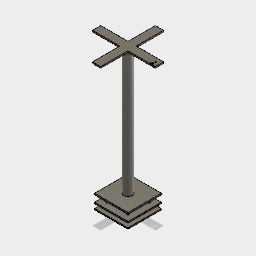
_FYP_Project.30689574-17b8-4f28-82bc-4a6d63cc6bb8 (Autodesk Fusion 360 design; units mm, degrees)
Autodesk Fusion 360 part; units mm, degrees
note: some values were not read from the file. Chosen so that the rebuilt part matches the saved one: which face or edge a step refers to. Set by a fixed rule: which sketch regions a step uses.
sketch "Sketch1" plane through (0, 0, 0) normal (1, 0, 0) x (0, 0, -1)
  circle A0 centre (0, 0) radius 40
  line L0 (-2.9, 1.75) -> (2.9, 1.75)
  line L1 (2.9, 1.75) -> (2.9, -1.75)
  line L2 (2.9, -1.75) -> (-2.9, -1.75)
  line L3 (-2.9, -1.75) -> (-2.9, 1.75)
  line L4 (-2.9, 1.75) -> (2.9, -1.75) construction
  line L5 (2.9, 1.75) -> (-2.9, -1.75) construction
  dimension "d1" = 80
  dimension "d2" = 5.8
  dimension "d3" = 3.5
  measures "d1" diameter of A0
  measures "d2" distance of L1.end L2.end
  measures "d3" distance of L0.end L1.end
sketch "Sketch2" plane through (0, 0, 0) normal (0, 1, 0) x (1, 0, 0)
  line L0 (16.6, 6) -> (-16.6, 6)
  line L1 (-16.6, 6) -> (-16.6, -6)
  line L2 (-16.6, -6) -> (16.6, -6)
  line L3 (16.6, -6) -> (16.6, 6)
  line L4 (16.6, 6) -> (-16.6, -6) construction
  line L5 (-16.6, 6) -> (16.6, -6) construction
  dimension "d6" = 33.2
  dimension "d7" = 12
  measures "d6" distance of L1.end L2.end
  measures "d7" distance of L0.end L1.end
extrude "Extrude2" add sketch "Sketch2" along normal blind 10 makes body 1
sketch "Sketch3" plane through (16.6, 0, 0) normal (1, 0, 0) x (0, 0, -1)
  line L0 (-6, 0) -> (6, 0)
  line L1 (6, 0) -> (6, 10)
  line L2 (6, 10) -> (-6, 10)
  line L3 (-6, 10) -> (-6, 0)
  circle A0 centre (-0.0016, 5.0186) radius 1.5
  line L4 (-1.2598, 5.8353) -> (1.2566, 5.8353)
  dimension "d10" = 3
  measures "d10" diameter of A0
extrude "Extrude3" add sketch "Sketch3" along normal blind 15 contours A0 L4 picked at (0.569, 4.736) bodies 1
sketch "Sketch4" plane through (0, 0, 0) normal (1, 0, 0) x (0, 0, -1)
  circle A0 centre (0, 0) radius 30
  dimension "d13" = 60
  measures "d13" diameter of A0
extrude "Extrude4" add sketch "Sketch4" along normal blind 8 separate body makes body 2
sketch "Sketch5" plane through (0, 0, 0) normal (-1, 0, 0) x (0, 0, 1)
  circle A0 centre (0, 0) radius 30
  circle A1 centre (0, 0) radius 1.5
  line L0 (-1.26, 0.8139) -> (1.26, 0.8139)
  dimension "d20" = 3
  dimension "d21" = 2.52
  measures "d20" diameter of A1
  measures "d21" distance of L0.start L0.end
extrude "Extrude5" cut sketch "Sketch5" against normal blind 14 contours A1 L0 picked at (-0.4465, 0.3176) bodies 2
copy_body "Body->Comp1" bodies 2 removing the originals makes body 3 in component "Component"
sketch "Sketch6" plane through (0, 0, 0) normal (0, 1, 0) x (1, 0, 0)
  line L0 (75, 100) -> (-75, 100)
  line L1 (-75, 100) -> (-75, -100)
  line L2 (-75, -100) -> (75, -100)
  line L3 (75, -100) -> (75, 100)
  line L4 (75, 100) -> (-75, -100) construction
  line L5 (-75, 100) -> (75, -100) construction
  dimension "d24" = 200
  dimension "d25" = 150
  measures "d24" distance of L0.end L1.end
  measures "d25" distance of L1.end L2.end
extrude "Extrude6" add sketch "Sketch6" along normal blind 6 separate body makes body 4
sketch "Sketch7" plane through (0, 6, 0) normal (0, 1, 0) x (-1, 0, 0)
  line L0 (-75, 100) -> (-75, -100)
  line L1 (-75, -100) -> (75, -100)
  line L2 (75, -100) -> (75, 100)
  line L3 (75, 100) -> (-75, 100)
  line L4 (-75, 38) -> (-41.8, 38)
  line L5 (-41.8, 38) -> (-41.8, 50)
  line L6 (-41.8, 50) -> (-75, 50)
  line L7 (-75, 50) -> (-75, 38)
  line L8 (-50.1369, 50) -> (-50.1369, 100)
  line L9 (75, 50) -> (41.8, 50)
  line L10 (41.8, 50) -> (41.8, 38)
  line L11 (41.8, 38) -> (75, 38)
  line L12 (75, 38) -> (75, 50)
  line L13 (63.0151, 50) -> (63.0151, 100)
  dimension "d28" = 33.2
  dimension "d29" = 12
  dimension "d30" = 50
  dimension "d31" = 33.2
  dimension "d32" = 12
  dimension "d33" = 50
  measures "d28" distance of L4.start L4.end
  measures "d29" distance of L4.start L6.end
  measures "d30" distance of L8.start L8.end
  measures "d31" distance of L9.start L9.end
  measures "d32" distance of L9.start L11.end
  measures "d33" distance of L13.start L13.end
extrude "Extrude7" add sketch "Sketch7" along normal blind 10 contours L0 L4 L5 L6 L7 | L2 L9 L10 L11 L12 bodies 4
sketch "Sketch8" plane through (75, 0, 0) normal (1, 0, 0) x (0, 0, -1)
  line L0 (-100, 0) -> (100, 0)
  line L1 (100, 0) -> (100, 6)
  line L2 (100, 6) -> (-38, 6)
  line L3 (-38, 6) -> (-38, 16)
  line L4 (-38, 16) -> (-50, 16)
  line L5 (-50, 16) -> (-50, 6)
  line L6 (-50, 6) -> (-100, 6)
  line L7 (-100, 6) -> (-100, 0)
  circle A0 centre (-44, 11) radius 1.5
  line L8 (-45.2778, 11.7856) -> (-42.7222, 11.7856)
  dimension "d36" = 3
  measures "d36" diameter of A0
extrude "Extrude8" add sketch "Sketch8" along normal blind 13 separate body contours A0 L8 | A0 L8 makes body 5
sketch "Sketch9" plane through (88, 0, 0) normal (1, 0, 0) x (0, 0, -1)
  circle A0 centre (-44, 11) radius 1.5
  line L0 (-42.8552, 11.9693) -> (-45.4152, 11.9693)
  dimension "d39" = 2.56
  measures "d39" distance of L0.start L0.end
extrude "Extrude9" cut sketch "Sketch9" against normal blind 17.5 contours A0 L0 picked at (-44.0921, 12.1771) bodies 4 5
sketch "Sketch10" plane through (88, 0, 0) normal (1, 0, 0) x (0, 0, -1)
  line L0 (-42.8552, 11.9693) -> (-45.1448, 11.9693)
  arc A0 (-45.1448, 11.9693) -> (-42.8552, 11.9693) centre (-44, 11) ccw
  circle A1 centre (-44, 11) radius 30
  dimension "d42" = 60
  measures "d42" diameter of A1
extrude "Extrude10" add sketch "Sketch10" against normal blind 6 bodies 5
move_face "OffsetFaces1" offset 2 1 faces at (88, 15.3388, 53.0097) on bodies 5
sketch "Sketch11" plane through (90, 0, 0) normal (1, 0, 0) x (0, 0, -1)
  circle A0 centre (-44, 11) radius 30
  circle A1 centre (-45.1448, 11.9693) radius 1.5
  point P0 (-45.1448, 11.9693)
  point P1 (-42.8552, 11.9693)
  dimension "d46" = 3
  measures "d46" diameter of A1
extrude "Extrude11" cut sketch "Sketch11" against normal blind 2 contours A1 bodies 5
sketch "Sketch12" plane through (-75, 0, 0) normal (-1, 0, 0) x (0, 0, 1)
  line L0 (-100, 0) -> (100, 0)
  line L1 (100, 0) -> (100, 6)
  line L2 (100, 6) -> (50, 6)
  line L3 (50, 6) -> (50, 16)
  line L4 (50, 16) -> (38, 16)
  line L5 (38, 16) -> (38, 6)
  line L6 (38, 6) -> (-100, 6)
  line L7 (-100, 6) -> (-100, 0)
  circle A0 centre (44, 11) radius 1.5
  line L8 (47.3889, 0) -> (45.2499, 0)
  line L9 (38.9976, 0) -> (40.5195, 0)
  dimension "d49" = 3
  measures "d49" diameter of A0
extrude "Extrude12" add sketch "Sketch12" along normal blind 13 contours A0 bodies 4
sketch "Sketch13" plane through (0, 16, 0) normal (0, 1, 0) x (-1, 0, 0)
  line L0 (-75, 50) -> (-75, 38)
  line L1 (-75, 38) -> (-41.8, 38)
  line L2 (-41.8, 38) -> (-41.8, 50)
  line L3 (-41.8, 50) -> (-75, 50)
sketch "Sketch14" plane through (-88, 0, 0) normal (-1, 0, 0) x (0, 0, 1)
  circle A0 centre (44, 11) radius 1.5
  line L0 (42.8552, 11.9693) -> (45.4152, 11.9693)
  point P0 (42.8552, 11.9693)
  dimension "d52" = 2.56
  measures "d52" distance of P0 L0.end
extrude "Extrude13" cut sketch "Sketch14" against normal blind 17 contours A0 L0 picked at (43.7391, 12.1515) bodies 4
sketch "Sketch15" plane through (-88, 0, 0) normal (-1, 0, 0) x (0, 0, 1)
  line L0 (45.1448, 11.9693) -> (42.8552, 11.9693)
  arc A0 (42.8552, 11.9693) -> (45.1448, 11.9693) centre (44, 11) ccw
  circle A1 centre (44, 11) radius 30
  dimension "d55" = 60
  measures "d55" diameter of A1
extrude "Extrude14" add sketch "Sketch15" along normal blind 8 separate body makes body 6
sketch "Sketch16" plane through (0, 6, 0) normal (0, 1, 0) x (-1, 0, 0)
  line L0 (-41.8, 38) -> (-75, 38)
  line L1 (-75, 38) -> (-75, -100)
  line L2 (-75, -100) -> (75, -100)
  line L3 (75, -100) -> (75, 38)
  line L4 (75, 38) -> (41.8, 38)
  line L5 (41.8, 38) -> (41.8, 50)
  line L6 (41.8, 50) -> (75, 50)
  line L7 (75, 50) -> (75, 100)
  line L8 (75, 100) -> (-75, 100)
  line L9 (-75, 100) -> (-75, 50)
  line L10 (-75, 50) -> (-41.8, 50)
  line L11 (-41.8, 50) -> (-41.8, 38)
  line L12 (-27.5, -85) -> (27.5, -85)
  line L13 (27.5, -85) -> (27.5, 85)
  line L14 (27.5, 85) -> (-27.5, 85)
  line L15 (-27.5, 85) -> (-27.5, -85)
  line L16 (-27.5, -85) -> (27.5, 85) construction
  line L17 (27.5, -85) -> (-27.5, 85) construction
  dimension "d58" = 170
  dimension "d59" = 55
  measures "d58" distance of L12.end L13.end
  measures "d59" distance of L13.end L14.end
extrude "Extrude15" add sketch "Sketch16" along normal blind 10 contours L12 L13 L14 L15 bodies 4
sketch "Sketch17" plane through (0, 6, 0) normal (0, 1, 0) x (-1, 0, 0)
  line L0 (-27.5, 85) -> (27.5, 85)
  line L1 (27.5, 85) -> (27.5, -85)
  line L2 (27.5, -85) -> (-27.5, -85)
  line L3 (-27.5, -85) -> (-27.5, 85)
  line L4 (-41.8, 38) -> (-75, 38)
  line L5 (-75, 38) -> (-75, -100)
  line L6 (-75, -100) -> (75, -100)
  line L7 (75, -100) -> (75, 38)
  line L8 (75, 38) -> (41.8, 38)
  line L9 (41.8, 38) -> (41.8, 50)
  line L10 (41.8, 50) -> (75, 50)
  line L11 (75, 50) -> (75, 100)
  line L12 (75, 100) -> (-75, 100)
  line L13 (-75, 100) -> (-75, 50)
  line L14 (-75, 50) -> (-41.8, 50)
  line L15 (-41.8, 50) -> (-41.8, 38)
  line L16 (75, 85) -> (60, 85)
  line L17 (60, 85) -> (60, 100)
  circle A0 centre (60, 85) radius 2.5
  dimension "d62" = 15
  dimension "d63" = 15
  dimension "d64" = 5
  measures "d62" distance of L16.start L16.end
  measures "d63" distance of L16.end L17.end
  measures "d64" diameter of A0
extrude "Extrude16" add sketch "Sketch17" along normal blind 40 contours L16 L17 A0 | L16 L17 A0 bodies 4
sketch "Sketch18" plane through (0, 6, 0) normal (0, 1, 0) x (-1, 0, 0)
  circle A0 centre (60, 85) radius 2.5
  line L0 (-27.5, 85) -> (27.5, 85)
  line L1 (27.5, 85) -> (27.5, -85)
  line L2 (27.5, -85) -> (-27.5, -85)
  line L3 (-27.5, -85) -> (-27.5, 85)
  line L4 (-41.8, 38) -> (-75, 38)
  line L5 (-75, 38) -> (-75, -100)
  line L6 (-75, -100) -> (75, -100)
  line L7 (75, -100) -> (75, 38)
  line L8 (75, 38) -> (41.8, 38)
  line L9 (41.8, 38) -> (41.8, 50)
  line L10 (41.8, 50) -> (75, 50)
  line L11 (75, 50) -> (75, 100)
  line L12 (75, 100) -> (-75, 100)
  line L13 (-75, 100) -> (-75, 50)
  line L14 (-75, 50) -> (-41.8, 50)
  line L15 (-41.8, 50) -> (-41.8, 38)
  line L16 (-60, 100) -> (-60, 85)
  line L17 (-60, 85) -> (-75, 85)
  circle A1 centre (-60, 85) radius 2.5
  dimension "d67" = 15
  dimension "d68" = 15
  dimension "d69" = 5
  measures "d67" distance of L16.start L16.end
  measures "d68" distance of L16.end L17.end
  measures "d69" diameter of A1
extrude "Extrude17" add sketch "Sketch18" along normal blind 40 contours L16 L17 A1 | L16 L17 A1 bodies 4
sketch "Sketch19" plane through (0, 6, 0) normal (0, 1, 0) x (-1, 0, 0)
  circle A0 centre (-60, 85) radius 2.5
  circle A1 centre (60, 85) radius 2.5
  line L0 (-27.5, 85) -> (27.5, 85)
  line L1 (27.5, 85) -> (27.5, -85)
  line L2 (27.5, -85) -> (-27.5, -85)
  line L3 (-27.5, -85) -> (-27.5, 85)
  line L4 (-41.8, 38) -> (-75, 38)
  line L5 (-75, 38) -> (-75, -100)
  line L6 (-75, -100) -> (75, -100)
  line L7 (75, -100) -> (75, 38)
  line L8 (75, 38) -> (41.8, 38)
  line L9 (41.8, 38) -> (41.8, 50)
  line L10 (41.8, 50) -> (75, 50)
  line L11 (75, 50) -> (75, 100)
  line L12 (75, 100) -> (-75, 100)
  line L13 (-75, 100) -> (-75, 50)
  line L14 (-75, 50) -> (-41.8, 50)
  line L15 (-41.8, 50) -> (-41.8, 38)
  line L16 (-60, -100) -> (-60, -85)
  line L17 (-60, -85) -> (-75, -85)
  circle A2 centre (-60, -85) radius 2.5
  dimension "d72" = 15
  dimension "d73" = 15
  dimension "d74" = 5
  measures "d72" distance of L16.end L17.end
  measures "d73" distance of L16.start L16.end
  measures "d74" diameter of A2
extrude "Extrude18" add sketch "Sketch19" along normal blind 40 contours L16 L17 A2 | L16 L17 A2 bodies 4
sketch "Sketch20" plane through (0, 6, 0) normal (0, 1, 0) x (-1, 0, 0)
  circle A0 centre (-60, -85) radius 2.5
  circle A1 centre (-60, 85) radius 2.5
  circle A2 centre (60, 85) radius 2.5
  line L0 (-27.5, 85) -> (27.5, 85)
  line L1 (27.5, 85) -> (27.5, -85)
  line L2 (27.5, -85) -> (-27.5, -85)
  line L3 (-27.5, -85) -> (-27.5, 85)
  line L4 (-41.8, 38) -> (-75, 38)
  line L5 (-75, 38) -> (-75, -100)
  line L6 (-75, -100) -> (75, -100)
  line L7 (75, -100) -> (75, 38)
  line L8 (75, 38) -> (41.8, 38)
  line L9 (41.8, 38) -> (41.8, 50)
  line L10 (41.8, 50) -> (75, 50)
  line L11 (75, 50) -> (75, 100)
  line L12 (75, 100) -> (-75, 100)
  line L13 (-75, 100) -> (-75, 50)
  line L14 (-75, 50) -> (-41.8, 50)
  line L15 (-41.8, 50) -> (-41.8, 38)
  line L16 (75, -85) -> (60, -85)
  line L17 (60, -85) -> (60, -100)
  circle A3 centre (60, -85) radius 2.5
  dimension "d77" = 15
  dimension "d78" = 15
  dimension "d79" = 5
  measures "d77" distance of L16.start L16.end
  measures "d78" distance of L16.end L17.end
  measures "d79" diameter of A3
extrude "Extrude19" add sketch "Sketch20" along normal blind 40 contours L16 L17 A3 | L16 L17 A3 bodies 4
sketch "Sketch21" plane through (0, 6, 0) normal (0, 1, 0) x (-1, 0, 0)
  circle A0 centre (60, -85) radius 2.5
  circle A1 centre (-60, -85) radius 2.5
  circle A2 centre (-60, 85) radius 2.5
  circle A3 centre (60, 85) radius 2.5
  line L0 (-27.5, 85) -> (27.5, 85)
  line L1 (27.5, 85) -> (27.5, -85)
  line L2 (27.5, -85) -> (-27.5, -85)
  line L3 (-27.5, -85) -> (-27.5, 85)
  line L4 (-41.8, 38) -> (-75, 38)
  line L5 (-75, 38) -> (-75, -100)
  line L6 (-75, -100) -> (75, -100)
  line L7 (75, -100) -> (75, 38)
  line L8 (75, 38) -> (41.8, 38)
  line L9 (41.8, 38) -> (41.8, 50)
  line L10 (41.8, 50) -> (75, 50)
  line L11 (75, 50) -> (75, 100)
  line L12 (75, 100) -> (-75, 100)
  line L13 (-75, 100) -> (-75, 50)
  line L14 (-75, 50) -> (-41.8, 50)
  line L15 (-41.8, 50) -> (-41.8, 38)
  line L16 (-75, 100) -> (-75, -100)
  line L17 (-75, 0) -> (-60, 0)
  circle A4 centre (-60, 0) radius 2.5
  dimension "d82" = 15
  dimension "d83" = 5
  measures "d82" distance of L17.start L17.end
  measures "d83" diameter of A4
extrude "Extrude20" add sketch "Sketch21" along normal blind 40 contours A4 bodies 4
sketch "Sketch22" plane through (0, 6, 0) normal (0, 1, 0) x (-1, 0, 0)
  circle A0 centre (-60, 0) radius 2.5
  circle A1 centre (60, -85) radius 2.5
  circle A2 centre (-60, -85) radius 2.5
  circle A3 centre (-60, 85) radius 2.5
  circle A4 centre (60, 85) radius 2.5
  line L0 (-27.5, 85) -> (27.5, 85)
  line L1 (27.5, 85) -> (27.5, -85)
  line L2 (27.5, -85) -> (-27.5, -85)
  line L3 (-27.5, -85) -> (-27.5, 85)
  line L4 (-41.8, 38) -> (-75, 38)
  line L5 (-75, 38) -> (-75, -100)
  line L6 (-75, -100) -> (75, -100)
  line L7 (75, -100) -> (75, 38)
  line L8 (75, 38) -> (41.8, 38)
  line L9 (41.8, 38) -> (41.8, 50)
  line L10 (41.8, 50) -> (75, 50)
  line L11 (75, 50) -> (75, 100)
  line L12 (75, 100) -> (-75, 100)
  line L13 (-75, 100) -> (-75, 50)
  line L14 (-75, 50) -> (-41.8, 50)
  line L15 (-41.8, 50) -> (-41.8, 38)
  line L16 (75, -100) -> (75, 100)
  line L17 (75, 0) -> (60, 0)
  circle A5 centre (60, 0) radius 2.5
  dimension "d86" = 15
  dimension "d87" = 5
  measures "d86" distance of L17.start L17.end
  measures "d87" diameter of A5
extrude "Extrude21" add sketch "Sketch22" along normal blind 40 contours A5 bodies 4
sketch "Sketch23" plane through (0, 46, 0) normal (0, 1, 0) x (-1, 0, 0)
  circle A0 centre (60, 85) radius 2.5
  line L0 (60, 85) -> (-59.9672, 85)
  line L1 (-59.9672, 85) -> (-59.9672, -85)
  line L2 (-59.9672, -85) -> (60, -85)
  line L3 (60, -85) -> (60, 85)
  line L4 (60, -85) -> (75, -85)
  line L5 (75, -85) -> (75, -100)
  line L6 (75, -100) -> (60, -100)
  line L7 (60, -100) -> (60, -85)
  line L8 (-59.9672, 85) -> (-75, 85)
  line L9 (-75, 85) -> (-75, 100)
  line L10 (-75, 100) -> (-59.9672, 100)
  line L11 (-59.9672, 100) -> (-59.9672, 85)
  line L12 (75, -100) -> (-75, -100)
  line L13 (-75, -100) -> (-75, 100)
  line L14 (-75, 100) -> (75, 100)
  line L15 (75, 100) -> (75, -100)
  point P0 (75, -100)
  point P1 (-75, 100)
extrude "Extrude22" add sketch "Sketch23" along normal blind 6 bodies 4
sketch "Sketch24" plane through (0, 52, 0) normal (0, 1, 0) x (-1, 0, 0)
  line L0 (75, 100) -> (-75, 100)
  line L1 (-75, 100) -> (-75, -100)
  line L2 (-75, -100) -> (75, -100)
  line L3 (75, -100) -> (75, 100)
  line L4 (75, 0) -> (60, 0)
  circle A0 centre (60, 0) radius 2.5
  dimension "d92" = 15
  dimension "d93" = 5
  measures "d92" distance of L4.start L4.end
  measures "d93" diameter of A0
extrude "Extrude23" add sketch "Sketch24" along normal blind 40 contours A0 bodies 4
sketch "Sketch25" plane through (0, 52, 0) normal (0, 1, 0) x (-1, 0, 0)
  circle A0 centre (60, 0) radius 2.5
  line L0 (75, 100) -> (-75, 100)
  line L1 (-75, 100) -> (-75, -100)
  line L2 (-75, -100) -> (75, -100)
  line L3 (75, -100) -> (75, 100)
  line L4 (-27.5, -85) -> (27.5, -85)
  line L5 (27.5, -85) -> (27.5, 85)
  line L6 (27.5, 85) -> (-27.5, 85)
  line L7 (-27.5, 85) -> (-27.5, -85)
  line L8 (-27.5, -85) -> (27.5, 85) construction
  line L9 (27.5, -85) -> (-27.5, 85) construction
  dimension "d96" = 170
  dimension "d97" = 55
  measures "d96" distance of L4.end L5.end
  measures "d97" distance of L5.end L6.end
extrude "Extrude24" add sketch "Sketch25" along normal blind 10 contours L4 L5 L6 L7 bodies 4
sketch "Sketch26" plane through (0, 52, 0) normal (0, 1, 0) x (-1, 0, 0)
  line L0 (-27.5, 85) -> (27.5, 85)
  line L1 (27.5, 85) -> (27.5, -85)
  line L2 (27.5, -85) -> (-27.5, -85)
  line L3 (-27.5, -85) -> (-27.5, 85)
  circle A0 centre (60, 0) radius 2.5
  line L4 (75, 100) -> (-75, 100)
  line L5 (-75, 100) -> (-75, -100)
  line L6 (-75, -100) -> (75, -100)
  line L7 (75, -100) -> (75, 100)
  line L8 (60, 100) -> (60, 85)
  line L9 (60, 85) -> (75, 85)
  circle A1 centre (60, 85) radius 2.5
  dimension "d100" = 15
  dimension "d101" = 15
  dimension "d102" = 5
  measures "d100" distance of L8.start L8.end
  measures "d101" distance of L8.end L9.end
  measures "d102" diameter of A1
extrude "Extrude25" add sketch "Sketch26" along normal blind 40 contours L8 L9 A1 | L8 L9 A1 bodies 4
sketch "Sketch27" plane through (0, 52, 0) normal (0, 1, 0) x (-1, 0, 0)
  circle A0 centre (60, 85) radius 2.5
  line L0 (-27.5, 85) -> (27.5, 85)
  line L1 (27.5, 85) -> (27.5, -85)
  line L2 (27.5, -85) -> (-27.5, -85)
  line L3 (-27.5, -85) -> (-27.5, 85)
  circle A1 centre (60, 0) radius 2.5
  line L4 (75, 100) -> (-75, 100)
  line L5 (-75, 100) -> (-75, -100)
  line L6 (-75, -100) -> (75, -100)
  line L7 (75, -100) -> (75, 100)
  line L8 (-54.2054, 100) -> (-54.2054, 78.5102)
  line L9 (-54.2054, 78.5102) -> (-75, 78.5102)
  circle A2 centre (-54.2054, 78.5102) radius 2.5
  dimension "d105" = 5
  measures "d105" diameter of A2
extrude "Extrude26" add sketch "Sketch27" along normal blind 40 contours L8 L9 A2 | L8 L9 A2 bodies 4
sketch "Sketch28" plane through (0, 52, 0) normal (0, 1, 0) x (-1, 0, 0)
  circle A0 centre (-54.2054, 78.5102) radius 2.5
  circle A1 centre (60, 85) radius 2.5
  line L0 (-27.5, 85) -> (27.5, 85)
  line L1 (27.5, 85) -> (27.5, -85)
  line L2 (27.5, -85) -> (-27.5, -85)
  line L3 (-27.5, -85) -> (-27.5, 85)
  circle A2 centre (60, 0) radius 2.5
  line L4 (75, 100) -> (-75, 100)
  line L5 (-75, 100) -> (-75, -100)
  line L6 (-75, -100) -> (75, -100)
  line L7 (75, -100) -> (75, 100)
  line L8 (-75, 0) -> (-60, 0)
  circle A3 centre (-60, 0) radius 2.5
  dimension "d108" = 15
  dimension "d109" = 5
  measures "d108" distance of L8.start L8.end
  measures "d109" diameter of A3
extrude "Extrude27" add sketch "Sketch28" along normal blind 40 contours A3 bodies 4
sketch "Sketch29" plane through (0, 52, 0) normal (0, 1, 0) x (-1, 0, 0)
  circle A0 centre (-60, 0) radius 2.5
  circle A1 centre (-54.2054, 78.5102) radius 2.5
  circle A2 centre (60, 85) radius 2.5
  line L0 (-27.5, 85) -> (27.5, 85)
  line L1 (27.5, 85) -> (27.5, -85)
  line L2 (27.5, -85) -> (-27.5, -85)
  line L3 (-27.5, -85) -> (-27.5, 85)
  circle A3 centre (60, 0) radius 2.5
  line L4 (75, 100) -> (-75, 100)
  line L5 (-75, 100) -> (-75, -100)
  line L6 (-75, -100) -> (75, -100)
  line L7 (75, -100) -> (75, 100)
  line L8 (-60, -100) -> (-60, -85)
  line L9 (-60, -85) -> (-75, -85)
  circle A4 centre (-60, -85) radius 2.5
  dimension "d112" = 15
  dimension "d113" = 15
  dimension "d114" = 5
  measures "d112" distance of L8.start L8.end
  measures "d113" distance of L8.end L9.end
  measures "d114" diameter of A4
extrude "Extrude28" add sketch "Sketch29" along normal blind 40 contours L8 L9 A4 | L8 L9 A4 bodies 4
sketch "Sketch30" plane through (0, 52, 0) normal (0, 1, 0) x (-1, 0, 0)
  circle A0 centre (-60, -85) radius 2.5
  circle A1 centre (-60, 0) radius 2.5
  circle A2 centre (-54.2054, 78.5102) radius 2.5
  circle A3 centre (60, 85) radius 2.5
  line L0 (-27.5, 85) -> (27.5, 85)
  line L1 (27.5, 85) -> (27.5, -85)
  line L2 (27.5, -85) -> (-27.5, -85)
  line L3 (-27.5, -85) -> (-27.5, 85)
  circle A4 centre (60, 0) radius 2.5
  line L4 (75, 100) -> (-75, 100)
  line L5 (-75, 100) -> (-75, -100)
  line L6 (-75, -100) -> (75, -100)
  line L7 (75, -100) -> (75, 100)
  line L8 (75, -85) -> (60, -85)
  line L9 (60, -85) -> (60, -100)
  circle A5 centre (60, -85) radius 2.5
  dimension "d117" = 15
  dimension "d118" = 15
  dimension "d119" = 5
  measures "d117" distance of L8.start L8.end
  measures "d118" distance of L8.end L9.end
  measures "d119" diameter of A5
extrude "Extrude29" add sketch "Sketch30" along normal blind 40 contours L8 L9 A5 | L8 L9 A5 bodies 4
sketch "Sketch31" plane through (0, 92, 0) normal (0, 1, 0) x (-1, 0, 0)
  circle A0 centre (60, -85) radius 2.5
  line L0 (60, -85) -> (-56.7054, -85)
  line L1 (-56.7054, -85) -> (-56.7054, 78.5102)
  line L2 (-56.7054, 78.5102) -> (60, 78.5102)
  line L3 (60, 78.5102) -> (60, -85)
  line L4 (60, -85) -> (75, -85)
  line L5 (75, -85) -> (75, -100)
  line L6 (75, -100) -> (60, -100)
  line L7 (60, -100) -> (60, -85)
  line L8 (75, -100) -> (-75, -100)
  line L9 (-75, -100) -> (-75, 100)
  line L10 (-75, 100) -> (75, 100)
  line L11 (75, 100) -> (75, -100)
  point P0 (-56.7054, 78.5102)
  point P1 (75, -100)
  point P2 (-75, 100)
extrude "Extrude30" add sketch "Sketch31" along normal blind 6 bodies 4
sketch "Sketch32" plane through (0, 98, 0) normal (0, 1, 0) x (-1, 0, 0)
  line L0 (75, 100) -> (-75, 100)
  line L1 (-75, 100) -> (-75, -100)
  line L2 (-75, -100) -> (75, -100)
  line L3 (75, -100) -> (75, 100)
  circle A0 centre (0, 0) radius 10
  dimension "d124" = 20
  measures "d124" diameter of A0
extrude "Extrude31" add sketch "Sketch32" along normal blind 60 contours A0 bodies 4
sphere "SpherePrimitive1" add diameter 50 placed x (-1, 0, 0) y (0, 0, 1) z (0, 1, 0) at (0, 158, 0) bodies 4
sketch "Sketch34" plane through (0, 98, 0) normal (0, 1, 0) x (-1, 0, 0)
  circle A0 centre (0, 0) radius 10
  line L0 (75, 100) -> (-75, 100)
  line L1 (-75, 100) -> (-75, -100)
  line L2 (-75, -100) -> (75, -100)
  line L3 (75, -100) -> (75, 100)
  line L4 (40, -40) -> (-40, -40)
  line L5 (-40, -40) -> (-40, 40)
  line L6 (-40, 40) -> (40, 40)
  line L7 (40, 40) -> (40, -40)
  line L8 (40, -40) -> (-40, 40) construction
  line L9 (-40, -40) -> (40, 40) construction
  circle A1 centre (0, 0) radius 20
  dimension "d128" = 80
  dimension "d129" = 80
  dimension "d130" = 40
  measures "d128" distance of L5.end L6.end
  measures "d129" distance of L4.end L5.end
  measures "d130" diameter of A1
extrude "Extrude32" add sketch "Sketch34" along normal blind 3 separate body contours L4 L5 L6 L7 makes body 7
sketch "Sketch35" plane through (0, 101, 0) normal (0, 1, 0) x (-1, 0, 0)
  circle A0 centre (0, 0) radius 20
  line L0 (40, 40) -> (-40, 40)
  line L1 (-40, 40) -> (-40, -40)
  line L2 (-40, -40) -> (40, -40)
  line L3 (40, -40) -> (40, 40)
  line L4 (25, 40) -> (25, 25)
  line L5 (25, 25) -> (40, 25)
  circle A1 centre (25, 25) radius 2.5
  dimension "d133" = 15
  dimension "d134" = 15
  dimension "d135" = 5
  measures "d133" distance of L4.start L4.end
  measures "d134" distance of L4.end L5.end
  measures "d135" diameter of A1
extrude "Extrude33" add sketch "Sketch35" along normal blind 10 contours L4 L5 A1 | L4 L5 A1 bodies 7
sketch "Sketch36" plane through (0, 101, 0) normal (0, 1, 0) x (-1, 0, 0)
  circle A0 centre (25, 25) radius 2.5
  circle A1 centre (0, 0) radius 20
  line L0 (40, 40) -> (-40, 40)
  line L1 (-40, 40) -> (-40, -40)
  line L2 (-40, -40) -> (40, -40)
  line L3 (40, -40) -> (40, 40)
  line L4 (25, -40) -> (25, -25)
  line L5 (25, -25) -> (40, -25)
  circle A2 centre (25, -25) radius 2.5
  dimension "d138" = 15
  dimension "d139" = 15
  dimension "d140" = 5
  measures "d138" distance of L4.end L5.end
  measures "d139" distance of L4.start L4.end
  measures "d140" diameter of A2
extrude "Extrude34" add sketch "Sketch36" along normal blind 10 contours L4 L5 A2 | L4 L5 A2 bodies 7
sketch "Sketch37" plane through (0, 101, 0) normal (0, 1, 0) x (-1, 0, 0)
  circle A0 centre (25, -25) radius 2.5
  circle A1 centre (25, 25) radius 2.5
  circle A2 centre (0, 0) radius 20
  line L0 (40, 40) -> (-40, 40)
  line L1 (-40, 40) -> (-40, -40)
  line L2 (-40, -40) -> (40, -40)
  line L3 (40, -40) -> (40, 40)
  line L4 (-25, -40) -> (-25, -25)
  line L5 (-25, -25) -> (-40, -25)
  circle A3 centre (-25, -25) radius 2.5
  dimension "d143" = 15
  dimension "d144" = 15
  dimension "d145" = 5
  measures "d143" distance of L4.start L4.end
  measures "d144" distance of L4.end L5.end
  measures "d145" diameter of A3
extrude "Extrude35" add sketch "Sketch37" along normal blind 10 contours L4 L5 A3 | L4 L5 A3 bodies 7
sketch "Sketch38" plane through (0, 101, 0) normal (0, 1, 0) x (-1, 0, 0)
  circle A0 centre (-25, -25) radius 2.5
  circle A1 centre (25, -25) radius 2.5
  circle A2 centre (25, 25) radius 2.5
  circle A3 centre (0, 0) radius 20
  line L0 (40, 40) -> (-40, 40)
  line L1 (-40, 40) -> (-40, -40)
  line L2 (-40, -40) -> (40, -40)
  line L3 (40, -40) -> (40, 40)
  line L4 (-25, 40) -> (-25, 25)
  line L5 (-25, 25) -> (-40, 25)
  circle A4 centre (-25, 25) radius 2.5
  dimension "d148" = 15
  dimension "d149" = 15
  dimension "d150" = 5
  measures "d148" distance of L4.start L4.end
  measures "d149" distance of L4.end L5.end
  measures "d150" diameter of A4
extrude "Extrude36" add sketch "Sketch38" along normal blind 10 contours L4 L5 A4 | L4 L5 A4 bodies 7
sketch "Sketch39" plane through (0, 111, 0) normal (0, 1, 0) x (-1, 0, 0)
  circle A0 centre (25, -25) radius 2.5
  line L0 (25, -25) -> (-25.2019, -25)
  line L1 (-25.2019, -25) -> (-25.2019, 25)
  line L2 (-25.2019, 25) -> (25, 25)
  line L3 (25, 25) -> (25, -25)
  line L4 (25, -25) -> (40, -25)
  line L5 (40, -25) -> (40, -40)
  line L6 (40, -40) -> (25, -40)
  line L7 (25, -40) -> (25, -25)
  line L8 (-25.2019, 25) -> (-40, 25)
  line L9 (-40, 25) -> (-40, 40)
  line L10 (-40, 40) -> (-25.2019, 40)
  line L11 (-25.2019, 40) -> (-25.2019, 25)
  line L12 (-40, 40) -> (40, 40)
  line L13 (40, 40) -> (40, -40)
  line L14 (40, -40) -> (-40, -40)
  line L15 (-40, -40) -> (-40, 40)
  point P0 (40, -40)
  point P1 (-40, 40)
extrude "Extrude37" add sketch "Sketch39" along normal blind 3 bodies 7
sketch "Sketch40" plane through (0, 114, 0) normal (0, 1, 0) x (-1, 0, 0)
  line L0 (-40, -40) -> (40, -40)
  line L1 (40, -40) -> (40, 40)
  line L2 (40, 40) -> (-40, 40)
  line L3 (-40, 40) -> (-40, -40)
  circle A0 centre (0, 0) radius 20
  dimension "d155" = 40
  measures "d155" diameter of A0
extrude "Extrude38" cut sketch "Sketch40" against normal blind 8 contours A0 bodies 7
sketch "Sketch41" plane through (0, 0, 0) normal (0, 1, 0) x (1, 0, 0)
sketch "Sketch42" plane through (0, 114, 0) normal (0, 1, 0) x (-1, 0, 0)
  circle A0 centre (0, 0) radius 20
  line L0 (-40, -40) -> (40, -40)
  line L1 (40, -40) -> (40, 40)
  line L2 (40, 40) -> (-40, 40)
  line L3 (-40, 40) -> (-40, -40)
  line L4 (40, 25) -> (25, 25)
  line L5 (25, 25) -> (25, 40)
  circle A1 centre (25, 25) radius 2.5
  dimension "d160" = 15
  dimension "d161" = 15
  dimension "d162" = 5
  measures "d160" distance of L4.start L4.end
  measures "d161" distance of L4.end L5.end
  measures "d162" diameter of A1
extrude "Extrude39" add sketch "Sketch42" along normal blind 15 contours L4 L5 A1 | L4 L5 A1 bodies 7
sketch "Sketch43" plane through (0, 114, 0) normal (0, 1, 0) x (-1, 0, 0)
  circle A0 centre (25, 25) radius 2.5
  circle A1 centre (0, 0) radius 20
  line L0 (-40, -40) -> (40, -40)
  line L1 (40, -40) -> (40, 40)
  line L2 (40, 40) -> (-40, 40)
  line L3 (-40, 40) -> (-40, -40)
  line L4 (-25, 40) -> (-25, 25)
  line L5 (-25, 25) -> (-40, 25.3183)
  circle A2 centre (-25, 25) radius 2.5
  dimension "d165" = 15
  dimension "d166" = 15
  dimension "d167" = 15
  dimension "d168" = 5
  measures "d165" distance of L4.start L4.end
  measures "d166" distance of L4.start L4.end
  measures "d167" distance of L4.end L5.end
  measures "d168" diameter of A2
extrude "Extrude40" add sketch "Sketch43" along normal blind 15 contours L4 L5 A2 | L4 L5 A2 bodies 7
sketch "Sketch44" plane through (0, 114, 0) normal (0, 1, 0) x (-1, 0, 0)
  circle A0 centre (-25, 25) radius 2.5
  circle A1 centre (25, 25) radius 2.5
  circle A2 centre (0, 0) radius 20
  line L0 (-40, -40) -> (40, -40)
  line L1 (40, -40) -> (40, 40)
  line L2 (40, 40) -> (-40, 40)
  line L3 (-40, 40) -> (-40, -40)
  line L4 (-25.5765, -40) -> (-25.5765, -25)
  line L5 (-25.5765, -25) -> (-40, -25)
  circle A3 centre (-25.5765, -25) radius 2.5
  dimension "d171" = 15
  dimension "d172" = 5
  measures "d171" distance of L4.start L4.end
  measures "d172" diameter of A3
extrude "Extrude41" add sketch "Sketch44" along normal blind 15 contours L4 L5 A3 | L4 L5 A3 bodies 7
sketch "Sketch45" plane through (0, 114, 0) normal (0, 1, 0) x (-1, 0, 0)
  circle A0 centre (-25.5765, -25) radius 2.5
  circle A1 centre (-25, 25) radius 2.5
  circle A2 centre (25, 25) radius 2.5
  circle A3 centre (0, 0) radius 20
  line L0 (-40, -40) -> (40, -40)
  line L1 (40, -40) -> (40, 40)
  line L2 (40, 40) -> (-40, 40)
  line L3 (-40, 40) -> (-40, -40)
  line L4 (25, -40) -> (25, -25)
  line L5 (25, -25) -> (40, -25)
  circle A4 centre (25, -25) radius 2.5
  dimension "d175" = 15
  dimension "d176" = 15
  dimension "d177" = 5
  measures "d175" distance of L4.end L5.end
  measures "d176" distance of L4.start L4.end
  measures "d177" diameter of A4
extrude "Extrude42" add sketch "Sketch45" along normal blind 15 contours L4 L5 A4 | L4 L5 A4 bodies 7
sketch "Sketch46" plane through (0, 129, 0) normal (0, 1, 0) x (-1, 0, 0)
  circle A0 centre (25, 25) radius 2.5
  line L0 (25, 25) -> (-25.7074, 25)
  line L1 (-25.7074, 25) -> (-25.7074, -24.951)
  line L2 (-25.7074, -24.951) -> (25, -24.951)
  line L3 (25, -24.951) -> (25, 25)
  line L4 (25, 25) -> (40, 25)
  line L5 (40, 25) -> (40, 40)
  line L6 (40, 40) -> (25, 40)
  line L7 (25, 40) -> (25, 25)
  line L8 (-25.7074, -24.951) -> (-40, -24.951)
  line L9 (-40, -24.951) -> (-40, -40)
  line L10 (-40, -40) -> (-25.7074, -40)
  line L11 (-25.7074, -40) -> (-25.7074, -24.951)
  line L12 (-40, -40) -> (40, -40)
  line L13 (40, -40) -> (40, 40)
  line L14 (40, 40) -> (-40, 40)
  line L15 (-40, 40) -> (-40, -40)
  point P0 (40, 40)
  point P1 (-40, -40)
extrude "Extrude43" add sketch "Sketch46" along normal blind 3.5 bodies 7
sketch "Sketch47" plane through (0, 0, 0) normal (1, 0, 0) x (0, 0, -1)
sketch "Sketch48" plane through (0, 132.5, 0) normal (0, 1, 0) x (-1, 0, 0)
  line L0 (-40, 40) -> (-40, -40)
  line L1 (-40, -40) -> (40, -40)
  line L2 (40, -40) -> (40, 40)
  line L3 (40, 40) -> (-40, 40)
  circle A0 centre (0, 0) radius 10
  dimension "d182" = 20
  measures "d182" diameter of A0
extrude "Extrude44" add sketch "Sketch48" along normal blind 300 contours A0 bodies 7
sketch "Sketch49" plane through (0, 432.5, 0) normal (0, 1, 0) x (-1, 0, 0)
  circle A0 centre (0, 0) radius 10
  line L0 (-75, -10) -> (75, -10)
  line L1 (75, -10) -> (75, 10)
  line L2 (75, 10) -> (-75, 10)
  line L3 (-75, 10) -> (-75, -10)
  line L4 (-75, -10) -> (75, 10) construction
  line L5 (75, -10) -> (-75, 10) construction
  line L6 (-10, -75) -> (10, -75)
  line L7 (10, -75) -> (10, 75)
  line L8 (10, 75) -> (-10, 75)
  line L9 (-10, 75) -> (-10, -75)
  line L10 (-10, -75) -> (10, 75) construction
  line L11 (10, -75) -> (-10, 75) construction
  dimension "d185" = 150
  dimension "d186" = 20
  dimension "d187" = 150
  dimension "d188" = 20
  measures "d185" distance of L1.end L2.end
  measures "d186" distance of L0.end L1.end
  measures "d187" distance of L6.end L7.end
  measures "d188" distance of L7.end L8.end
extrude "Extrude45" add sketch "Sketch49" along normal blind 3.5 bodies 7
sketch "Sketch50" plane through (0, 436, 0) normal (0, 1, 0) x (-1, 0, 0)
  line L0 (-10, 75) -> (-10, 10)
  line L1 (-10, 10) -> (-75, 10)
  line L2 (-75, 10) -> (-75, -10)
  line L3 (-75, -10) -> (-10, -10)
  line L4 (-10, -10) -> (-10, -75)
  line L5 (-10, -75) -> (10, -75)
  line L6 (10, -75) -> (10, -10)
  line L7 (10, -10) -> (75, -10)
  line L8 (75, -10) -> (75, 10)
  line L9 (75, 10) -> (10, 10)
  line L10 (10, 10) -> (10, 75)
  line L11 (10, 75) -> (-10, 75)
  line L12 (-66.1169, 0) -> (-66.1169, 9)
  line L13 (-66.1169, 0) -> (-63.7875, 8.6933)
  line L14 (-66.1169, 0) -> (-61.6169, 7.7942)
  circle A0 centre (-66.1169, 0) radius 1.5
  line L15 (-61.9584, 7.7027) -> (-64.2084, 3.8056)
  arc A1 (-64.2084, 3.8056) -> (-63.7754, 3.5556) centre (-63.9919, 3.6806) ccw
  line L16 (-63.7754, 3.5556) -> (-61.5254, 7.4527)
  arc A2 (-61.5254, 7.4527) -> (-61.9584, 7.7027) centre (-61.7419, 7.5777) ccw
  line L17 (-61.6169, 7.7942) -> (-64.1169, 3.4641) construction
  line L18 (-64.0937, 8.5166) -> (-65.2584, 4.1699)
  arc A3 (-65.2584, 4.1699) -> (-64.7754, 4.0405) centre (-65.0169, 4.1052) ccw
  line L19 (-64.7754, 4.0405) -> (-63.6107, 8.3871)
  arc A4 (-63.6107, 8.3871) -> (-64.0937, 8.5166) centre (-63.8522, 8.4519) ccw
  line L20 (-63.7875, 8.6933) -> (-65.0816, 3.8637) construction
  line L21 (-66.3669, 8.75) -> (-66.3669, 4.25)
  arc A5 (-66.3669, 4.25) -> (-65.8669, 4.25) centre (-66.1169, 4.25) ccw
  line L22 (-65.8669, 4.25) -> (-65.8669, 8.75)
  arc A6 (-65.8669, 8.75) -> (-66.3669, 8.75) centre (-66.1169, 8.75) ccw
  line L23 (-66.1169, 9) -> (-66.1169, 4) construction
  dimension "d196" = 9
  dimension "d197" = 9
  dimension "d198" = 15
  dimension "d199" = 9
  dimension "d200" = 15
  dimension "d201" = 3
  dimension "d202" = 0.5
  dimension "d203" = 0.5
  dimension "d204" = 0.5
  measures "d196" distance of L12.start L12.end
  measures "d197" distance of L12.start L13.end
  measures "d198" angle of L12 L13
  measures "d199" distance of L12.start L14.end
  measures "d200" angle of L13 L14
  measures "d201" diameter of A0
  measures "d202" diameter of A1
  measures "d203" diameter of A3
  measures "d204" diameter of A5
extrude "Extrude46" cut sketch "Sketch50" against normal blind 3.5 contours L12 L14 A0 | L12 L13 A0 | L13 L14 A0 | L12 L21 A5 A6 | L12 A5 L22 A6 | L13 L18 A3 A4 | L13 A3 L19 A4 | L14 L15 A1 A2 | L14 A1 L16 A2 bodies 7
sketch "Sketch51" plane through (0, 6, 0) normal (0, 1, 0) x (-1, 0, 0)
  circle A0 centre (60, 0) radius 2.5
  circle A1 centre (-60, 0) radius 2.5
  circle A2 centre (60, -85) radius 2.5
  circle A3 centre (-60, -85) radius 2.5
  circle A4 centre (-60, 85) radius 2.5
  circle A5 centre (60, 85) radius 2.5
  line L0 (-27.5, 85) -> (27.5, 85)
  line L1 (27.5, 85) -> (27.5, -85)
  line L2 (27.5, -85) -> (-27.5, -85)
  line L3 (-27.5, -85) -> (-27.5, 85)
  line L4 (-41.8, 38) -> (-75, 38)
  line L5 (-75, 38) -> (-75, -100)
  line L6 (-75, -100) -> (75, -100)
  line L7 (75, -100) -> (75, 38)
  line L8 (75, 38) -> (41.8, 38)
  line L9 (41.8, 38) -> (41.8, 50)
  line L10 (41.8, 50) -> (75, 50)
  line L11 (75, 50) -> (75, 100)
  line L12 (75, 100) -> (-75, 100)
  line L13 (-75, 100) -> (-75, 50)
  line L14 (-75, 50) -> (-41.8, 50)
  line L15 (-41.8, 50) -> (-41.8, 38)
  line L16 (-32.5, -95) -> (-42.5, -95)
  line L17 (-42.5, -95) -> (-42.5, -65)
  line L18 (-42.5, -65) -> (-32.5, -65)
  line L19 (-32.5, -65) -> (-32.5, -95)
  line L20 (32.5, -65) -> (42.5, -65)
  line L21 (42.5, -65) -> (42.5, -95)
  line L22 (42.5, -95) -> (32.5, -95)
  line L23 (32.5, -95) -> (32.5, -65)
  dimension "d207" = 10
  dimension "d208" = 30
  dimension "d209" = 5
  dimension "d210" = 5
  dimension "d211" = 10
  dimension "d212" = 30
  dimension "d213" = 5
  dimension "d214" = 5
  measures "d207" distance of L16.start L16.end
  measures "d208" distance of L16.start L18.end
  measures "d209" distance of L6 L16
  measures "d210" distance of L3 L19
  measures "d211" distance of L20.start L20.end
  measures "d212" distance of L20.start L22.end
  measures "d213" distance of L6 L22
  measures "d214" distance of L1 L23
extrude "Extrude47" add sketch "Sketch51" against normal blind 11 contours L16 L17 L18 L19 | L20 L21 L22 L23 bodies 4
move_face "OffsetFaces2" offset 5 2 faces at (35.8333, -1.6667, -95) (-39.1667, -1.6667, -95) on bodies 4
sketch "Sketch52" plane through (0, 0, -100) normal (0, 0, -1) x (-1, 0, 0)
  line L0 (-42.5, 0) -> (-42.5, -5)
  line L1 (-42.5, -5) -> (-32.5, -5)
  line L2 (-32.5, -5) -> (-32.5, 0)
  line L3 (-32.5, 0) -> (32.5, 0)
  line L4 (32.5, 0) -> (32.5, -5)
  line L5 (32.5, -5) -> (42.5, -5)
  line L6 (42.5, -5) -> (42.5, 0)
  line L7 (42.5, 0) -> (75, 0)
  line L8 (75, 0) -> (75, 6)
  line L9 (75, 6) -> (-75, 6)
  line L10 (-75, 6) -> (-75, 0)
  line L11 (-75, 0) -> (-42.5, 0)
  line L12 (-42.5, -5) -> (-32.5, -5)
  line L13 (-32.5, -5) -> (-32.5, 6)
  line L14 (-32.5, 6) -> (-42.5, 6)
  line L15 (-42.5, 6) -> (-42.5, -5)
  dimension "d218" = 11
  dimension "d219" = 10
  measures "d218" distance of L0.end L14.end
  measures "d219" distance of L0.end L1.end
extrude "Extrude48" add sketch "Sketch52" along normal blind 5 contours L0 L1 L2 L9 L12 L13 L14 L15 bodies 4
sketch "Sketch53" plane through (0, 0, -100) normal (0, 0, -1) x (-1, 0, 0)
  line L0 (-32.5, 6) -> (-32.5, 0)
  line L1 (-32.5, 0) -> (32.5, 0)
  line L2 (32.5, 0) -> (32.5, -5)
  line L3 (32.5, -5) -> (42.5, -5)
  line L4 (42.5, -5) -> (42.5, 0)
  line L5 (42.5, 0) -> (75, 0)
  line L6 (75, 0) -> (75, 6)
  line L7 (75, 6) -> (-32.5, 6)
  line L8 (32.5, -5) -> (42.5, -5)
  line L9 (42.5, -5) -> (42.5, 6)
  line L10 (42.5, 6) -> (32.5, 6)
  line L11 (32.5, 6) -> (32.5, -5)
  dimension "d222" = 10
  measures "d222" distance of L2.end L3.end
extrude "Extrude49" add sketch "Sketch53" along normal blind 5 contours L2 L3 L4 L7 L8 L9 L10 L11 bodies 4
sketch "Sketch54" plane through (0, 0, -85) normal (0, 0, -1) x (-1, 0, 0)
  line L0 (-27.5, 6) -> (27.5, 6)
  line L1 (27.5, 6) -> (27.5, 16)
  line L2 (27.5, 16) -> (-27.5, 16)
  line L3 (-27.5, 16) -> (-27.5, 6)
  line L4 (-42.5, 6) -> (42.5, 6)
  line L5 (42.5, 6) -> (42.5, -5)
  line L6 (42.5, -5) -> (-42.5, -5)
  line L7 (-42.5, -5) -> (-42.5, 6)
  point P0 (-42.5, 6)
  point P1 (42.5, -5)
extrude "Extrude50" add sketch "Sketch54" along normal blind 20 contours L0 L4 L5 L6 L7 bodies 4
move_face "OffsetFaces3" offset -19 1 faces at (10.8333, -3.3333, -85) on bodies 4
sketch "Sketch55" plane through (0, 6, 0) normal (0, 1, 0) x (-1, 0, 0)
  line L0 (-27.5, -85) -> (-27.5, 85)
  line L1 (-27.5, 85) -> (27.5, 85)
  line L2 (27.5, 85) -> (27.5, -85)
  line L3 (27.5, -85) -> (-27.5, -85)
  circle A0 centre (60, 85) radius 2.5
  circle A1 centre (-60, 85) radius 2.5
  circle A2 centre (-60, -85) radius 2.5
  circle A3 centre (60, -85) radius 2.5
  circle A4 centre (-60, 0) radius 2.5
  circle A5 centre (60, 0) radius 2.5
  line L4 (-42.5, -105) -> (42.5, -105)
  line L5 (42.5, -105) -> (42.5, -100)
  line L6 (42.5, -100) -> (75, -100)
  line L7 (75, -100) -> (75, 38)
  line L8 (75, 38) -> (41.8, 38)
  line L9 (41.8, 38) -> (41.8, 50)
  line L10 (41.8, 50) -> (75, 50)
  line L11 (75, 50) -> (75, 100)
  line L12 (75, 100) -> (-75, 100)
  line L13 (-75, 100) -> (-75, 50)
  line L14 (-75, 50) -> (-41.8, 50)
  line L15 (-41.8, 50) -> (-41.8, 38)
  line L16 (-41.8, 38) -> (-75, 38)
  line L17 (-75, 38) -> (-75, -100)
  line L18 (-75, -100) -> (-42.5, -100)
  line L19 (-42.5, -100) -> (-42.5, -105)
move_face "OffsetFaces4" offset 5 1 faces at (-14.1667, -1.3333, -105) on bodies 4
sketch "Sketch56" plane through (0, -5, 0) normal (0, -1, 0) x (1, 0, 0)
  line L0 (42.5, -110) -> (42.5, -65)
  line L1 (42.5, -65) -> (32.5, -65)
  line L2 (32.5, -65) -> (32.5, -104)
  line L3 (32.5, -104) -> (-32.5, -104)
  line L4 (-32.5, -104) -> (-32.5, -65)
  line L5 (-32.5, -65) -> (-42.5, -65)
  line L6 (-42.5, -65) -> (-42.5, -110)
  line L7 (-42.5, -110) -> (42.5, -110)
  line L8 (-42.5, -110) -> (-32.5, -110)
  line L9 (-32.5, -110) -> (-32.5, -104)
  line L10 (-32.5, -104) -> (-42.5, -104)
  line L11 (-42.5, -104) -> (-42.5, -110)
  line L12 (42.5, -110) -> (32.5, -110)
  line L13 (32.5, -110) -> (32.5, -104)
  line L14 (32.5, -104) -> (42.5, -104)
  line L15 (42.5, -104) -> (42.5, -110)
extrude "Extrude51" add sketch "Sketch56" along normal blind 10 contours L0 L7 L12 L13 L14 L15 | L6 L7 L8 L9 L10 L11 bodies 4
move_face "OffsetFaces5" offset -10 1 faces at (10.8333, -5, -106) on bodies 4
sketch "Sketch57" plane through (32.5, 0, 0) normal (-1, 0, 0) x (0, 0, 1)
  line L0 (-104, 5) -> (-110, 5)
  line L1 (-110, 5) -> (-110, -15)
  line L2 (-110, -15) -> (-104, -15)
  line L3 (-104, -15) -> (-104, -5)
  line L4 (-104, -5) -> (-65, -5)
  line L5 (-65, -5) -> (-65, 0)
  line L6 (-65, 0) -> (-104, 0)
  line L7 (-104, 0) -> (-104, 5)
  circle A0 centre (-107, -11) radius 7.5
  dimension "d232" = 15
  dimension "d233" = 5
  dimension "d234" = 5
  measures "d232" diameter of A0
  measures "d233" distance of L2.end A0.centre
  measures "d234" distance of L1.end A0.centre
extrude "Extrude52" add sketch "Sketch57" along normal blind 65 contours L1 L2 L3 L4 A0 | L1 L2 L3 L4 A0 bodies 4
sketch "Sketch58" plane through (0, 0, 0) normal (0, 1, 0) x (1, 0, 0)
component "Component" placed x (1, 0, 0) y (0, 1, 0) z (0, 0, 1) at (0, 0, 0)
hidden bodies 1 4 5 6 3
